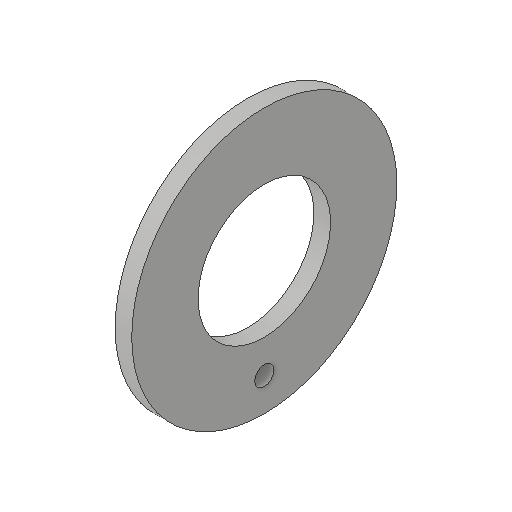
# Autodesk Inventor part: SKF_PCMW 122401.5 E
Saved by Autodesk Inventor 2022 (Build 260153000, 153)
## iProperties
Category: PARTsolutions
Company: SKF
Created: 2022-07-25
Part Number: SKF_PCMW 122401.5 E
Material: Generic
Catalog Web Link: www.cadenas.de
Description: BPT_001-Thrust washers
Vendor: SKF
Document SubType Name: Modeling
Designer: psAdmin
Manufacturer: SKF
Mass: 3.8 g
Surface Area: 8.51666 cm^2
Volume: 0.50533 cm^3
Density: 1 g/cm^3
Appearance: PSOLRGB-175-175-175
PSOL_IDENT_0: {$CADENAS_DATA/23d-libs/skf/bearings_units_and_housings/plain_bearings/bushings_washers_and_strips/b
PSOL_IDENT_1: pt_001.prj},180 {VTYP=3D},{NB=SKF_PCMW 122401.5 E},{LINA=SKF_PCMW 122401.5 E},{NN=BPT_001},{DATE=08.
PSOL_IDENT_2: 07.2022 10:25:42},{GEOMDATE=16.02.2021 08:39:09},{VERSION=},{LINEID=900},{WBVAR=},{WBNUMERIC=}  {NB=
PSOL_IDENT_3: SKF_PCMW 122401.5 E},{LINA=SKF_PCMW 122401.5 E},{KT=DUMMY},{DESIGNATION=PCMW 122401.5 E},{DD=12.000}
PSOL_IDENT_4: ,{D=24.000},{H=1.500},{J=18.000},{K=1.750},{DA=24},{JA=18},{HA=1.0},{LOAD1=28.000},{LOAD2=85.000},{L
PSOL_IDENT_5: OAD3=80},{LOAD4=250},{KM=300},{VMAX=2},{VMIN=0},{MIMAX=0.25},{MIMIN=0.03},{MASS=0.0038},{A=},{POPULA
PSOL_IDENT_6: R=}
NB: SKF_PCMW 122401.5 E
NN: BPT_001
NT: Thrust washers
NBSYN: SKF_$DESIGNATION.
LINA: SKF_PCMW 122401.5 E
CATALOG: SKF
DESIGNATION: PCMW 122401.5 E
DD: 12
D: 24
H: 1.5
LOAD1: 28
LOAD2: 85
SUPPLIER: SKF
ARTICLENO: SKF_PCMW 122401.5 E
BOMINFO: SKF_PCMW 122401.5 E
CREATOR: CADENAS GmbH
Title: SKF_PCMW 122401.5 E
Author: Cadenas PARTsolutions
Comments: Thrust washers
Autodesk Inventor part; units mm, degrees
ref_plane "YZ Plane" through (0, 0, 0) normal (1, 0, 0) x (0, 1, 0)
ref_plane "XZ Plane" through (0, 0, 0) normal (0, 1, 0) x (-1, 0, 0)
ref_plane "XY Plane" through (0, 0, 0) normal (0, 0, 1) x (1, 0, 0)
sketch "Sketch_1" plane through (0, 0, 0) normal (0, 0, 1) x (1, 0, 0)
  line L0 (1.5, 0) -> (-1.5, 0)
  line L1 (0, 12) -> (0, 6)
  line L2 (0, 6) -> (1.5, 6)
  line L3 (1.5, 6) -> (1.5, 12)
  line L4 (1.5, 12) -> (0, 12)
  constraints: 10 end point
revolve "Revolution1" add sketch "Sketch_1" angle 360 about axis through (1.5, 0, 0) along (1, 0, 0)
sketch "Sketch2" plane through (0, 0, 0) normal (-1, 0, 0) x (0, 0, 1)
  point P0 (0, -9)
hole "Hole1" at (0, -9, 0) direction (1, 0, 0) diameter 1.75 depth 1.5
body "Solid1"
